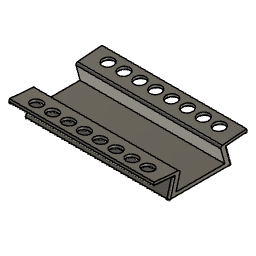
PCRtubeMagnetHolder v3 (Autodesk Fusion 360 design; units mm, degrees)
Autodesk Fusion 360 part; units mm, degrees
note: some values were not read from the file. Set by a fixed rule: which sketch regions a step uses.
sketch "Sketch1" plane through (0, 0, 0) normal (1, 0, 0) x (0, 1, 0)
  line L0 (15.3144, 0) -> (15.3144, 3)
  line L1 (15.3144, 3) -> (29.1526, 3)
  line L2 (29.1526, 3) -> (26.5644, 12.6593)
  line L3 (29.1526, 3) -> (39.1526, 3) construction
  line L4 (26.5644, 12.6593) -> (41.5073, 13.9666)
  line L5 (26.5644, 12.6593) -> (41.5644, 12.6593) construction
  line L6 (41.5073, 13.9666) -> (42.1544, 11.5518)
  line L7 (33.588, 0) -> (30.7598, 10.5549)
  line L8 (42.1544, 11.5518) -> (30.7598, 10.5549)
  line L9 (33.588, 0) -> (15.3144, 0)
  dimension "d2" = 3
  dimension "d7" = 105
  dimension "d8" = 10
  dimension "d9" = 5
  dimension "d10" = 15
  dimension "d11" = 2.5
  dimension "d73" = 11.25
  constraint perpendicular L0 L1
  constraint horizontal L3
  constraint horizontal L5
  constraint parallel L2 L6
  constraint parallel L2 L7
  constraint parallel L4 L8
  constraint perpendicular L0 L9
  measures "d2" distance of L0.start L0.end
  measures "d7" angle of L2 L3
  measures "d8" distance of L1.end L2.end
  measures "d9" angle of L4 L5
  measures "d10" distance of L2.end L4.end
  measures "d11" distance of L4.end L6.end
  measures "d73" horizontal distance of L0.end L2.end
extrude "Extrude1" add sketch "Sketch1" against normal blind 82
sketch "Sketch3" plane through (0, -0.8973, 10.2567) normal (0, -0.087156, 0.996195) x (1, 0, 0)
  line L0 (0, 27.5666) -> (0, 42.5666)
  line L1 (0, 42.5666) -> (-82, 42.5666)
  line L2 (-82, 42.5666) -> (-82, 27.5666)
  line L3 (-82, 27.5666) -> (0, 27.5666)
  line L4 (-82, 42.5666) -> (-82, 36.5666) construction
  line L5 (-82, 36.5666) -> (0, 36.5666)
  circle A0 centre (-72.5, 36.5666) radius 3.25
  circle A1 centre (-45.5, 36.5666) radius 3.25
  circle A2 centre (-54.5, 36.5666) radius 3.25
  circle A3 centre (-63.5, 36.5666) radius 3.25
  circle A4 centre (-9.5, 36.5596) radius 3.25
  circle A5 centre (-18.5, 36.5596) radius 3.25
  circle A6 centre (-27.5, 36.5666) radius 3.25
  circle A7 centre (-36.5, 36.5666) radius 3.25
  dimension "d21" = 6
  dimension "d31" = 6.5
  dimension "d34" = 6.5
  dimension "d35" = 6.5
  dimension "d37" = 9
  dimension "d39" = 6.5
  dimension "d43" = 6.5
  dimension "d44" = 6.5
  dimension "d45" = 6.5
  dimension "d46" = 6.5
  dimension "d47" = 9
  dimension "d48" = 9
  dimension "d49" = 9
  dimension "d50" = 9
  dimension "d52" = 9
  dimension "d53" = 9
  dimension "d78" = 9.5
  dimension "d80" = 9.5
  constraint coincident L1.end L2.start
  constraint perpendicular L1 L4
  constraint coincident L0 L5.end
  constraint perpendicular L0 L5
  measures "d21" distance of L1.end L4.end
  measures "d34" diameter of A1
  measures "d35" diameter of A2
  measures "d37" distance of A1.centre A2.centre
  measures "d39" diameter of A3
  measures "d43" diameter of A7
  measures "d44" diameter of A6
  measures "d45" diameter of A4
  measures "d46" diameter of A5
  measures "d47" distance of A4.centre A5.centre
  measures "d48" distance of A1.centre A7.centre
  measures "d49" distance of A7.centre A6.centre
  measures "d50" distance of A6.centre A5.centre
  measures "d52" distance of A2.centre A3.centre
  measures "d53" distance of A0.centre A3.centre
  measures "d78" distance of L4 A0.centre
  measures "d80" distance of L0 A4.centre
extrude "Extrude2" cut sketch "Sketch3" against normal blind 2.5 contours L5 A4 | L5 A4 | L5 A0 | L5 A0 | L5 A5 | L5 A5 | L5 A3 | L5 A3 | L5 A6 | L5 A6 | L5 A2 | L5 A2 | L5 A7 | L5 A7 | L5 A1 | L5 A1
mirror "Mirror1" about plane through (0, 15.3144, 0) normal (0, -1, 0) of bodies 1 merged
fillet "Fillet3" radius 1 16 edges at (-41, 26.5644, 12.6593) (-41, 4.0644, 12.6593) (-41, -2.9592, 0) (-82, -1.5451, 5.2774) (-82, 32.1739, 5.2774) (-41, 33.588, 0) (0, 15.3144, 0) (-82, 15.3144, 0) (-82, 36.4571, 11.0533) (-41, 42.1544, 11.5518) (0, 36.4571, 11.0533) (0, -5.8283, 11.0533) (0, 32.1739, 5.2774) (0, -1.5451, 5.2774) (-41, -11.5256, 11.5518) (-82, -5.8283, 11.0533)
fillet "Fillet4" radius 1 16 edges at (-75.5301, 34.5739, 10.8886) (-66.5301, 34.5739, 10.8886) (-57.5301, 34.5739, 10.8886) (-48.5301, 34.5739, 10.8886) (-39.5301, 34.5739, 10.8886) (-30.5301, 34.5739, 10.8886) (-21.5301, 34.5669, 10.888) (-12.5301, 34.5669, 10.888) (-75.5301, -3.9452, 10.8886) (-66.5301, -3.9452, 10.8886) (-57.5301, -3.9452, 10.8886) (-48.5301, -3.9452, 10.8886) (-39.5301, -3.9452, 10.8886) (-30.5301, -3.9452, 10.8886) (-21.5301, -3.9381, 10.888) (-12.5301, -3.9381, 10.888)
